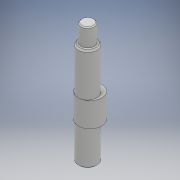
# Autodesk Inventor part: 도면2-4번
Saved by Autodesk Inventor 2018.3 (Build 223284000, 284)
## iProperties
Created: 2019-10-11
Part Number: 도면2-4번
Material: 일반
Document SubType Name: Modeling
Designer: MyTool
Density: 1 g/cm^3
Appearance: 기본값
Author: MyTool
Autodesk Inventor part; units mm, degrees
ref_plane "YZ Plane" through (0, 0, 0) normal (1, 0, 0) x (0, 1, 0)
ref_plane "XZ Plane" through (0, 0, 0) normal (0, 1, 0) x (-1, 0, 0)
ref_plane "XY Plane" through (0, 0, 0) normal (0, 0, 1) x (1, 0, 0)
sketch "스케치1" plane through (0, 0, 0) normal (1, 0, 0) x (0, 1, 0)
  line L0 (0, 0) -> (10, 0)
  line L1 (10, 0) -> (10, 37)
  line L2 (10, 37) -> (0, 37)
  line L3 (0, 37) -> (0, 0)
  line L4 (0, 37) -> (15, 37)
  line L5 (15, 37) -> (15, 63)
  line L6 (15, 63) -> (0, 63)
  line L7 (0, 63) -> (0, 37)
  line L8 (0, 63) -> (10, 63)
  line L9 (10, 63) -> (10, 109)
  line L10 (10, 109) -> (0, 109)
  line L11 (0, 109) -> (0, 63)
  line L12 (0, 109) -> (7, 109)
  line L13 (7, 109) -> (7, 128)
  line L14 (7, 128) -> (0, 128)
  line L15 (0, 128) -> (0, 109)
  dimension "d1" = 37
  dimension "d2" = 26
  dimension "d3" = 46
  dimension "d4" = 20
  dimension "d5" = 30
  dimension "d6" = 19
  dimension "d7" = 14
  constraints: 32 end point, 8 parallel, 4 horizontal, 4 perpendicular, 1 collinear
  measures "d1" distance of L0.end L1.end
  measures "d2" distance of L4.end L5.end
  measures "d3" distance of L8.end L9.end
  measures "d4" diameter of L1 L3
  measures "d5" diameter of L5 L7
  measures "d6" distance of L12.end L13.end
  measures "d7" diameter of L13 L15
revolve "회전1" add sketch "스케치1" angle 360 about axis through (0, 0, 63) along (0, 0, -1)
sketch "스케치2" plane through (0, 0, 63) normal (0, 0, 1) x (1, 0, 0)
  circle A0 centre (0, 0) radius 10 projected
  circle A1 centre (0, 2.5) radius 12.5
  circle A2 centre (0, 0) radius 15 projected
  point P0 (0, 0)
  dimension "d9" = 25
  constraints: 1 centre point, 1 tangent
  measures "d9" diameter of A1
sketch "스케치2 outline for 돌출1" plane through (0, 0, 63) normal (0, 0, 1) x (1, 0, 0)
  arc A0 (0, 15) -> (15, 0) centre (0, 0) ccw
  arc A1 (15, 0) -> (0, 15) centre (0, 0) ccw
  arc A2 (0, 15) -> (12.5, 2.5) centre (0, 2.5) ccw
  arc A3 (12.5, 2.5) -> (0, 15) centre (0, 2.5) ccw
extrude "돌출1" cut sketch "스케치2 outline for 돌출1" against normal up to next
sketch "스케치3" plane through (0, 0, 0) normal (1, 0, 0) x (0, 1, 0)
  line L0 (10, 109) -> (10, 63)
  line L1 (-10, 109) -> (10, 109)
  line L2 (10, 109) -> (10, 107.008142)
  line L3 (8.85, 109) -> (10, 109)
  line L4 (8.85, 109) -> (10, 107.008142)
  line L5 (0, -21.8) -> (0, 130.8)
  point P0 (0, 0)
  dimension "d12" = 30
  dimension "d13" = 1.15
  constraints: 6 end point, 1 perpendicular, 1 point on line
  measures "d12" angle of L4 L0
  measures "d13" distance of L0.start L3.start
revolve "회전2" cut sketch "스케치3" angle 360 about axis through (0, 0, -10) along (0, 0, 1)
sketch "스케치4" plane through (0, 0, 0) normal (0, 0, -1) x (-1, 0, 0)
  circle A0 centre (0, 0) radius 1.5
  dimension "d15" = 3
  constraints: 1 centre point, 1 coincident
  measures "d15" diameter of A0
hole "구멍1" at (0, 0, 0) direction (0, 0, 1) diameter 2.459 depth 11.5 tip angle 118 thread size "M3x0.5" class "6H" standard "ANSI Metric M Profile"
sketch "스케치6" plane through (0, 0, 0) normal (0, 1, 0) x (-1, 0, 0)
  line L0 (7, 128) -> (7, 109) projected
  line L1 (7, 114) -> (4, 114)
  line L2 (4, 114) -> (4, 124)
  line L3 (4, 124) -> (7, 124)
  line L4 (7, 114) -> (7, 124)
  point P0 (0, 0)
  dimension "d29" = 4
  dimension "d30" = 10
  dimension "d31" = 3
  constraints: 8 end point, 3 perpendicular, 2 point on line, 1 horizontal
  measures "d29" distance from line of L0.start L3
  measures "d30" distance of L1.end L2.end
  measures "d31" distance of L1.start L1.end
extrude "돌출3" cut sketch "스케치6" along normal mid plane 5
fillet "모깎기2" radius 2.5 4 edges at (-5.2692, 2.5, 114) (-5.2692, -2.5, 114) (-5.2692, 2.5, 124) (-5.2692, -2.5, 124)
sketch "스케치8" plane through (0, 0, 0) normal (1, 0, 0) x (0, 1, 0)
  line L0 (7, 128) -> (7, 109) projected
  line L1 (7, 112) -> (6, 112)
  line L2 (6, 112) -> (7, 113)
  line L3 (7, 112) -> (7, 113)
  point P0 (0, 0)
  dimension "d35" = 45
  dimension "d36" = 1
  dimension "d37" = 3
  constraints: 6 end point, 2 point on line, 1 perpendicular
  measures "d35" angle of L2 L1
  measures "d36" distance of L2.end L1.start
  measures "d37" distance of L1.start L0.end
revolve "회전3" cut sketch "스케치8" angle 360 about axis through (0, 7, 112) along (0, -1, 0)
chamfer "모따기1" distance 1 angle 45 2 edges at (0, -7, 128) (0, -10, 0)
